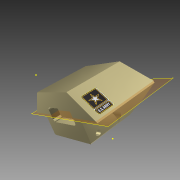
# Autodesk Inventor part: Correct BACK PIECE
Saved by Autodesk Inventor 2015 (Build 190159000, 159)
## iProperties
Created: 2015-04-17
Part Number: Correct BACK PIECE
Material: Generic
Document SubType Name: Modeling
Designer: Simrun
Density: 1 g/cm^3
Appearance: Gold - Metal
Mass: 1012.93 g
Surface Area: 682.37 cm^2
Volume: 1012.93 cm^3
Author: Simrun
Autodesk Inventor part; units mm, degrees
ref_plane "YZ Plane" through (0, 0, 0) normal (1, 0, 0) x (0, 1, 0)
ref_plane "XZ Plane" through (0, 0, 0) normal (0, 1, 0) x (-1, 0, 0)
sketch "Sketch1" plane through (0, 0, 0) normal (0, 0, 1) x (1, 0, 0)
  line L0 (0, 0) -> (0, 77.724)
  line L1 (0, 77.724) -> (101.6, 77.724)
  line L2 (101.6, 77.724) -> (114.3, 38.862)
  line L3 (114.3, 38.862) -> (101.6, 17.4625)
  line L4 (101.6, 17.4625) -> (92.075, 7.9375)
  line L5 (92.075, 7.9375) -> (79.375, 0)
  line L6 (79.375, 0) -> (0, 0)
  dimension "d0" = 77.724
  dimension "d1" = 101.6
  constraints: 14 end point, 1 horizontal, 1 perpendicular, 1 vertical
  measures "d0" distance of L0.start L0.end
  measures "d1" distance of L0.end L1.end
extrude "Extrusion1" add sketch "Sketch1" against normal blind 171.45
chamfer "Chamfer1" distance 41.275 angle 45 1 edges at (50.8, 77.724, 0)
chamfer "Chamfer2" distance 36.449 angle 45 1 edges at (39.6875, 0, 0)
chamfer "Chamfer3" distance 41.275 angle 45 1 edges at (50.8, 77.724, -171.45)
chamfer "Chamfer4" distance 36.449 angle 45 1 edges at (39.6875, 0, -171.45)
ref_plane "Work Plane1" through (0, 122.174, -85.725) normal (0, 0, 1) x (1, 0, 0)
ref_plane "Work Plane2" through (0, 0, -35.052) normal (0, 0, 1) x (1, 0, 0)
sketch "Sketch2" plane through (0, 0, -35.052) normal (0, 0, 1) x (1, 0, 0)
  line L0 (0, 36.449) -> (0, 0) projected
  line L1 (0, 1.5875) -> (0, 36.5125)
  line L2 (0, 36.5125) -> (19.2786, 36.5125)
  line L3 (0, 0) -> (79.375, 0) projected
  arc A0 (54.1154, 0) -> (19.2786, 36.5125) centre (19.2786, 1.6373) ccw
  line L4 (0, 1.5875) -> (54.1538, 1.5875)
  dimension "d17" = 34.925
  dimension "d18" = 19.2786
  constraints: 6 end point, 3 point on circle, 2 point on line, 1 centre point, 1 collinear, 1 parallel, 1 perpendicular, 1 tangent
  measures "d17" distance of L1.start L1.end
  measures "d18" distance of L1.end L2.end
extrude "Extrusion2" add sketch "Sketch2" along normal blind 35.052 contours L1 L2 A0 L4 L0
sketch "Sketch3" plane through (0, 0, 0) normal (0, 0, 1) x (1, 0, 0)
  line L0 (0, 1.5875) -> (0, 36.5125)
  line L1 (0, 77.724) -> (0, 36.5125) projected
  line L2 (0, 36.5125) -> (19.2786, 36.5125)
  line L3 (0, 36.5125) -> (19.2786, 36.5125) projected
  arc A0 (55.5625, 1.5875) -> (19.2786, 36.5125) centre (20.2634, 1.2253) ccw
  line L4 (55.5625, 1.5875) -> (0, 1.5875)
  line L5 (0, 0) -> (79.375, 0) projected
  constraints: 6 end point, 2 collinear, 2 point on circle, 1 centre point, 1 parallel
extrude "Extrusion3" cut sketch "Sketch3" against normal blind 35.052
mirror "Mirror1" about plane through (0, 122.174, -85.725) normal (0, 0, 1) of "Extrusion3"
ref_plane "Work Plane3" through (112.868, 36.449, 0) normal (-0.0005626, -0.9999998, 0) x (-0.9999997, 0.0005626, -0.0005626)
sketch "Sketch4" plane through (0, 0, -35.052) normal (0, 0, 1) x (1, 0, 0)
  line L0 (55.5625, 1.5875) -> (16.6624, 1.5875)
  line L1 (55.5625, 1.5875) -> (0, 1.5875) projected
  line L2 (16.6624, 1.5875) -> (16.6624, 7.9375)
  circle A0 centre (16.6624, 7.9375) radius 4.572
  point P0 (0, 0)
  dimension "d23" = 38.9001
  dimension "d24" = 6.35
  dimension "d25" = 9.144
  constraints: 4 end point, 1 centre point, 1 coincident, 1 point on line, 1 vertical
  measures "d23" distance of L0.start L0.end
  measures "d24" distance of L0.end L2.end
  measures "d25" diameter of A0
extrude "Extrusion4" cut sketch "Sketch4" against normal blind 10.16
mirror "Mirror2" about plane through (0, 122.174, -85.725) normal (0, 0, 1) of "Extrusion4"
sketch "Sketch5" plane through (0, 77.724, -41.275) normal (0, 0.7071068, 0.7071068) x (1, 0, 0)
  line L0 (10.4166, -16.3549) -> (37.5444, -16.3549) construction
  line L1 (37.5444, -16.3549) -> (37.5444, -50.6938) construction
  line L2 (37.5444, -50.6938) -> (10.4166, -50.6938) construction
  line L3 (10.4166, -50.6938) -> (10.4166, -16.3549) construction
  point P0 (0, -84.145)
  constraints: 2 other
sketch "Sketch6" plane through (0, 77.724, -130.175) normal (-1, 0, 0) x (0, 0, 1)
  line L0 (12.7, -26.162) -> (76.2, -26.162)
  line L1 (76.2, -26.162) -> (76.2, -51.562)
  line L2 (76.2, -51.562) -> (12.7, -51.562)
  line L3 (12.7, -51.562) -> (12.7, -26.162)
  line L4 (95.123, -76.1365) -> (95.123, -41.2115) projected
  line L5 (88.9, 0) -> (0, 0) projected
  point P0 (130.175, -77.724)
  dimension "d44" = 63.5
  dimension "d45" = 25.4
  dimension "d46" = 18.923
  dimension "d47" = 26.162
  constraints: 8 end point, 2 horizontal, 2 perpendicular
  measures "d44" distance of L0.start L0.end
  measures "d45" distance of L0.end L1.end
  measures "d46" distance between parallel lines of L4 L1
  measures "d47" distance between parallel lines of L5 L0
extrude "Extrusion5" cut sketch "Sketch6" against normal blind 14.478
fillet "Fillet1" radius 5.08 4 edges at (7.239, 51.562, -117.475) (7.239, 51.562, -53.975) (7.239, 26.162, -117.475) (7.239, 26.162, -53.975)
ref_plane "Work Plane4" through (0, 38.862, -41.275) normal (0, 1, 0) x (1, 0, 0)
sketch "Sketch7" plane through (114.3, 38.862, -2.413) normal (0.9505306, 0.3106309, 0) x (0, 0, -1)
  line L0 (68.5999, 25.7598) -> (96.6605, 25.7598) construction
  line L1 (96.6605, 25.7598) -> (96.6605, 14.7456) construction
  line L2 (96.6605, 14.7456) -> (68.5999, 14.7456) construction
  line L3 (68.5999, 14.7456) -> (68.5999, 25.7598) construction
  line L4 (71.7776, 31.7341) -> (71.0108, 31.7341)
  line L5 (71.0108, 31.7341) -> (69.7861, 33.9468)
  line L6 (69.7861, 33.9468) -> (69.7861, 31.7341)
  line L7 (69.7861, 31.7341) -> (69.058, 31.7341)
  line L8 (69.058, 31.7341) -> (69.058, 34.9091)
  line L9 (69.058, 34.9091) -> (70.0357, 34.9091)
  line L10 (70.0357, 34.9091) -> (71.0494, 33.0901)
  line L11 (71.0494, 33.0901) -> (71.0494, 34.9091)
  line L12 (71.0494, 34.9091) -> (71.7776, 34.9091)
  line L13 (71.7776, 34.9091) -> (71.7776, 31.7341)
  line L14 (72.4234, 31.7341) -> (72.4234, 34.9091)
  line L15 (72.4234, 34.9091) -> (74.5692, 34.9091)
  line L16 (74.5692, 34.9091) -> (74.5692, 34.3045)
  line L17 (74.5692, 34.3045) -> (73.2158, 34.3045)
  line L18 (73.2158, 34.3045) -> (73.2158, 33.7462)
  line L19 (73.2158, 33.7462) -> (74.4637, 33.7462)
  line L20 (74.4637, 33.7462) -> (74.4637, 33.1415)
  line L21 (74.4637, 33.1415) -> (73.2158, 33.1415)
  line L22 (73.2158, 33.1415) -> (73.2158, 32.3388)
  line L23 (73.2158, 32.3388) -> (74.5692, 32.3388)
  line L24 (74.5692, 32.3388) -> (74.5692, 31.7341)
  line L25 (74.5692, 31.7341) -> (72.4234, 31.7341)
  line L26 (77.7596, 34.9091) -> (76.6687, 31.7341)
  line L27 (76.6687, 31.7341) -> (75.8377, 31.7341)
  line L28 (75.8377, 31.7341) -> (74.7467, 34.9091)
  line L29 (74.7467, 34.9091) -> (75.5726, 34.9091)
  line L30 (75.5726, 34.9091) -> (76.2648, 32.7556)
  line L31 (76.2648, 32.7556) -> (76.9543, 34.9091)
  line L32 (76.9543, 34.9091) -> (77.7596, 34.9091)
  line L33 (78.0555, 31.7341) -> (78.0555, 34.9091)
  line L34 (78.0555, 34.9091) -> (80.2014, 34.9091)
  line L35 (80.2014, 34.9091) -> (80.2014, 34.3045)
  line L36 (80.2014, 34.3045) -> (78.848, 34.3045)
  line L37 (78.848, 34.3045) -> (78.848, 33.7462)
  line L38 (78.848, 33.7462) -> (80.0959, 33.7462)
  line L39 (80.0959, 33.7462) -> (80.0959, 33.1415)
  line L40 (80.0959, 33.1415) -> (78.848, 33.1415)
  line L41 (78.848, 33.1415) -> (78.848, 32.3388)
  line L42 (78.848, 32.3388) -> (80.2014, 32.3388)
  line L43 (80.2014, 32.3388) -> (80.2014, 31.7341)
  line L44 (80.2014, 31.7341) -> (78.0555, 31.7341)
  line L45 (83.6748, 31.7341) -> (82.7048, 31.7341)
  line L46 (82.7048, 31.7341) -> (81.8223, 32.8997)
  line L47 (81.8223, 32.8997) -> (81.5341, 32.8997)
  line L48 (81.5341, 32.8997) -> (81.5341, 31.7341)
  line L49 (81.5341, 31.7341) -> (80.7417, 31.7341)
  line L50 (80.7417, 31.7341) -> (80.7417, 34.9091)
  line L51 (80.7417, 34.9091) -> (82.0178, 34.9091)
  spline S0 degree 2 poles (82.0178, 34.9091) (82.2829, 34.9091) (82.6739, 34.8422) (82.8412, 34.7393) knots 0 0 0 1 2 2 2
  spline S1 degree 2 poles (82.8412, 34.7393) (83.011, 34.6312) (83.2117, 34.2942) (83.2117, 34.0369) knots 0 0 0 1 2 2 2
  spline S2 degree 2 poles (83.2117, 34.0369) (83.2117, 33.6741) (82.8823, 33.2187) (82.607, 33.0849) knots 0 0 0 1 2 2 2
  line L52 (82.607, 33.0849) -> (83.6748, 31.7341)
  spline S3 degree 2 poles (82.3935, 33.9366) (82.3935, 34.0575) (82.3009, 34.2299) (82.1954, 34.2762) knots 0 0 0 1 2 2 2
  spline S4 degree 2 poles (82.1954, 34.2762) (82.1208, 34.3071) (81.9381, 34.3251) (81.8017, 34.3251) knots 0 0 0 1 2 2 2
  line L53 (81.8017, 34.3251) -> (81.5341, 34.3251)
  line L54 (81.5341, 34.3251) -> (81.5341, 33.4709)
  line L55 (81.5341, 33.4709) -> (81.7631, 33.4709)
  spline S5 degree 2 poles (81.7631, 33.4709) (81.9278, 33.4709) (82.1619, 33.512) (82.2417, 33.5763) knots 0 0 0 1 2 2 2
  spline S6 degree 2 poles (82.2417, 33.5763) (82.3189, 33.6381) (82.3935, 33.8028) (82.3935, 33.9366) knots 0 0 0 1 2 2 2
  spline S7 degree 2 poles (86.1706, 31.6775) (85.8052, 31.6775) (85.2546, 31.819) (85.0179, 31.9219) knots 0 0 0 1 2 2 2
  line L56 (85.0179, 31.9219) -> (85.0179, 32.6784)
  line L57 (85.0179, 32.6784) -> (85.0899, 32.6784)
  spline S8 degree 2 poles (85.0899, 32.6784) (85.3292, 32.4751) (85.903, 32.2564) (86.1731, 32.2564) knots 0 0 0 1 2 2 2
  spline S9 degree 2 poles (86.1731, 32.2564) (86.2426, 32.2564) (86.4664, 32.2873) (86.5333, 32.3182) knots 0 0 0 1 2 2 2
  spline S10 degree 2 poles (86.5333, 32.3182) (86.6157, 32.3542) (86.7315, 32.4854) (86.7315, 32.5909) knots 0 0 0 1 2 2 2
  spline S11 degree 2 poles (86.7315, 32.5909) (86.7315, 32.7118) (86.5436, 32.8611) (86.415, 32.8945) knots 0 0 0 1 2 2 2
  spline S12 degree 2 poles (86.415, 32.8945) (86.2529, 32.9383) (85.885, 33.0129) (85.7229, 33.0695) knots 0 0 0 1 2 2 2
  spline S13 degree 2 poles (85.7229, 33.0695) (85.3549, 33.1981) (85.0359, 33.6381) (85.0359, 33.9674) knots 0 0 0 1 2 2 2
  spline S14 degree 2 poles (85.0359, 33.9674) (85.0359, 34.4125) (85.7898, 34.9657) (86.3558, 34.9657) knots 0 0 0 1 2 2 2
  spline S15 degree 2 poles (86.3558, 34.9657) (86.6388, 34.9657) (87.1997, 34.8499) (87.421, 34.7522) knots 0 0 0 1 2 2 2
  line L58 (87.421, 34.7522) -> (87.421, 34.0266)
  line L59 (87.421, 34.0266) -> (87.3515, 34.0266)
  spline S16 degree 2 poles (87.3515, 34.0266) (87.174, 34.1784) (86.6646, 34.3868) (86.397, 34.3868) knots 0 0 0 1 2 2 2
  spline S17 degree 2 poles (86.397, 34.3868) (86.2915, 34.3868) (86.1268, 34.3559) (86.0342, 34.3148) knots 0 0 0 1 2 2 2
  spline S18 degree 2 poles (86.0342, 34.3148) (85.9596, 34.2813) (85.8515, 34.1475) (85.8515, 34.0652) knots 0 0 0 1 2 2 2
  spline S19 degree 2 poles (85.8515, 34.0652) (85.8515, 33.9417) (86.0239, 33.8002) (86.2709, 33.7436) knots 0 0 0 1 2 2 2
  spline S20 degree 2 poles (86.2709, 33.7436) (86.4304, 33.7076) (86.7263, 33.6381) (86.8961, 33.5789) knots 0 0 0 1 2 2 2
  spline S21 degree 2 poles (86.8961, 33.5789) (87.2255, 33.458) (87.5471, 33.0566) (87.5471, 32.7273) knots 0 0 0 1 2 2 2
  spline S22 degree 2 poles (87.5471, 32.7273) (87.5471, 32.2539) (86.8035, 31.6775) (86.1706, 31.6775) knots 0 0 0 1 2 2 2
  line L60 (88.566, 31.7341) -> (88.566, 34.3045)
  line L61 (88.566, 34.3045) -> (87.6268, 34.3045)
  line L62 (87.6268, 34.3045) -> (87.6268, 34.9091)
  line L63 (87.6268, 34.9091) -> (90.3027, 34.9091)
  line L64 (90.3027, 34.9091) -> (90.3027, 34.3045)
  line L65 (90.3027, 34.3045) -> (89.3636, 34.3045)
  line L66 (89.3636, 34.3045) -> (89.3636, 31.7341)
  line L67 (89.3636, 31.7341) -> (88.566, 31.7341)
  spline S23 degree 2 poles (93.5189, 33.3216) (93.5189, 32.5497) (92.6955, 31.6672) (91.9802, 31.6672) knots 0 0 0 1 2 2 2
  spline S24 degree 2 poles (91.9802, 31.6672) (91.2624, 31.6672) (90.4442, 32.56) (90.4442, 33.3216) knots 0 0 0 1 2 2 2
  spline S25 degree 2 poles (90.4442, 33.3216) (90.4442, 34.0858) (91.2624, 34.976) (91.9802, 34.976) knots 0 0 0 1 2 2 2
  spline S26 degree 2 poles (91.9802, 34.976) (92.6955, 34.976) (93.5189, 34.0909) (93.5189, 33.3216) knots 0 0 0 1 2 2 2
  spline S27 degree 2 poles (92.6955, 33.3216) (92.6955, 33.6072) (92.5797, 34.006) (92.4794, 34.1321) knots 0 0 0 1 2 2 2
  spline S28 degree 2 poles (92.4794, 34.1321) (92.379, 34.2633) (92.1218, 34.3765) (91.9828, 34.3765) knots 0 0 0 1 2 2 2
  spline S29 degree 2 poles (91.9828, 34.3765) (91.8362, 34.3765) (91.5969, 34.271) (91.4862, 34.1372) knots 0 0 0 1 2 2 2
  spline S30 degree 2 poles (91.4862, 34.1372) (91.3885, 34.0137) (91.2675, 33.6046) (91.2675, 33.3216) knots 0 0 0 1 2 2 2
  spline S31 degree 2 poles (91.2675, 33.3216) (91.2675, 33.0283) (91.3833, 32.6424) (91.4837, 32.5111) knots 0 0 0 1 2 2 2
  spline S32 degree 2 poles (91.4837, 32.5111) (91.584, 32.3799) (91.8439, 32.2667) (91.9828, 32.2667) knots 0 0 0 1 2 2 2
  spline S33 degree 2 poles (91.9828, 32.2667) (92.1243, 32.2667) (92.3868, 32.3876) (92.482, 32.5163) knots 0 0 0 1 2 2 2
  spline S34 degree 2 poles (92.482, 32.5163) (92.5849, 32.6552) (92.6955, 33.0232) (92.6955, 33.3216) knots 0 0 0 1 2 2 2
  spline S35 degree 2 poles (96.434, 33.9082) (96.434, 33.687) (96.2925, 33.2856) (96.1613, 33.1518) knots 0 0 0 1 2 2 2
  spline S36 degree 2 poles (96.1613, 33.1518) (96.0815, 33.0669) (95.886, 32.928) (95.7702, 32.8791) knots 0 0 0 1 2 2 2
  spline S37 degree 2 poles (95.7702, 32.8791) (95.6518, 32.8302) (95.3765, 32.7736) (95.2067, 32.7736) knots 0 0 0 1 2 2 2
  line L68 (95.2067, 32.7736) -> (94.7899, 32.7736)
  line L69 (94.7899, 32.7736) -> (94.7899, 31.7341)
  line L70 (94.7899, 31.7341) -> (93.9923, 31.7341)
  line L71 (93.9923, 31.7341) -> (93.9923, 34.9091)
  line L72 (93.9923, 34.9091) -> (95.2247, 34.9091)
  spline S38 degree 2 poles (95.2247, 34.9091) (95.4974, 34.9091) (95.8962, 34.8088) (96.0583, 34.7007) knots 0 0 0 1 2 2 2
  spline S39 degree 2 poles (96.0583, 34.7007) (96.2384, 34.5798) (96.434, 34.1836) (96.434, 33.9082) knots 0 0 0 1 2 2 2
  spline S40 degree 2 poles (95.6158, 33.8877) (95.6158, 34.024) (95.4872, 34.217) (95.3997, 34.253) knots 0 0 0 1 2 2 2
  spline S41 degree 2 poles (95.3997, 34.253) (95.2865, 34.3019) (95.0806, 34.3173) (94.9031, 34.3173) knots 0 0 0 1 2 2 2
  line L73 (94.9031, 34.3173) -> (94.7899, 34.3173)
  line L74 (94.7899, 34.3173) -> (94.7899, 33.3654)
  line L75 (94.7899, 33.3654) -> (94.8465, 33.3654)
  spline S42 degree 2 poles (94.8465, 33.3654) (94.9571, 33.3654) (95.1578, 33.3705) (95.2324, 33.3834) knots 0 0 0 1 2 2 2
  spline S43 degree 2 poles (95.2324, 33.3834) (95.2968, 33.3937) (95.4383, 33.4554) (95.4769, 33.494) knots 0 0 0 1 2 2 2
  spline S44 degree 2 poles (95.4769, 33.494) (95.5592, 33.5712) (95.6158, 33.7436) (95.6158, 33.8877) knots 0 0 0 1 2 2 2
  line L76 (78.2524, 21.279) -> (77.4856, 21.279)
  line L77 (77.4856, 21.279) -> (76.2609, 23.4917)
  line L78 (76.2609, 23.4917) -> (76.2609, 21.279)
  line L79 (76.2609, 21.279) -> (75.5328, 21.279)
  line L80 (75.5328, 21.279) -> (75.5328, 24.454)
  line L81 (75.5328, 24.454) -> (76.5105, 24.454)
  line L82 (76.5105, 24.454) -> (77.5242, 22.6349)
  line L83 (77.5242, 22.6349) -> (77.5242, 24.454)
  line L84 (77.5242, 24.454) -> (78.2524, 24.454)
  line L85 (78.2524, 24.454) -> (78.2524, 21.279)
  line L86 (78.8982, 21.279) -> (78.8982, 24.454)
  line L87 (78.8982, 24.454) -> (81.044, 24.454)
  line L88 (81.044, 24.454) -> (81.044, 23.8494)
  line L89 (81.044, 23.8494) -> (79.6906, 23.8494)
  line L90 (79.6906, 23.8494) -> (79.6906, 23.291)
  line L91 (79.6906, 23.291) -> (80.9385, 23.291)
  line L92 (80.9385, 23.291) -> (80.9385, 22.6864)
  line L93 (80.9385, 22.6864) -> (79.6906, 22.6864)
  line L94 (79.6906, 22.6864) -> (79.6906, 21.8837)
  line L95 (79.6906, 21.8837) -> (81.044, 21.8837)
  line L96 (81.044, 21.8837) -> (81.044, 21.279)
  line L97 (81.044, 21.279) -> (78.8982, 21.279)
  line L98 (84.2344, 24.454) -> (83.1435, 21.279)
  line L99 (83.1435, 21.279) -> (82.3124, 21.279)
  line L100 (82.3124, 21.279) -> (81.2215, 24.454)
  line L101 (81.2215, 24.454) -> (82.0474, 24.454)
  line L102 (82.0474, 24.454) -> (82.7396, 22.3005)
  line L103 (82.7396, 22.3005) -> (83.4291, 24.454)
  line L104 (83.4291, 24.454) -> (84.2344, 24.454)
  line L105 (84.5303, 21.279) -> (84.5303, 24.454)
  line L106 (84.5303, 24.454) -> (86.6761, 24.454)
  line L107 (86.6761, 24.454) -> (86.6761, 23.8494)
  line L108 (86.6761, 23.8494) -> (85.3228, 23.8494)
  line L109 (85.3228, 23.8494) -> (85.3228, 23.291)
  line L110 (85.3228, 23.291) -> (86.5706, 23.291)
  line L111 (86.5706, 23.291) -> (86.5706, 22.6864)
  line L112 (86.5706, 22.6864) -> (85.3228, 22.6864)
  line L113 (85.3228, 22.6864) -> (85.3228, 21.8837)
  line L114 (85.3228, 21.8837) -> (86.6761, 21.8837)
  line L115 (86.6761, 21.8837) -> (86.6761, 21.279)
  line L116 (86.6761, 21.279) -> (84.5303, 21.279)
  line L117 (90.1496, 21.279) -> (89.1796, 21.279)
  line L118 (89.1796, 21.279) -> (88.2971, 22.4446)
  line L119 (88.2971, 22.4446) -> (88.0089, 22.4446)
  line L120 (88.0089, 22.4446) -> (88.0089, 21.279)
  line L121 (88.0089, 21.279) -> (87.2165, 21.279)
  line L122 (87.2165, 21.279) -> (87.2165, 24.454)
  line L123 (87.2165, 24.454) -> (88.4926, 24.454)
  spline S45 degree 2 poles (88.4926, 24.454) (88.7576, 24.454) (89.1487, 24.3871) (89.316, 24.2842) knots 0 0 0 1 2 2 2
  spline S46 degree 2 poles (89.316, 24.2842) (89.4858, 24.1761) (89.6865, 23.8391) (89.6865, 23.5818) knots 0 0 0 1 2 2 2
  spline S47 degree 2 poles (89.6865, 23.5818) (89.6865, 23.219) (89.3571, 22.7636) (89.0818, 22.6298) knots 0 0 0 1 2 2 2
  line L124 (89.0818, 22.6298) -> (90.1496, 21.279)
  spline S48 degree 2 poles (88.8683, 23.4814) (88.8683, 23.6024) (88.7757, 23.7748) (88.6702, 23.8211) knots 0 0 0 1 2 2 2
  spline S49 degree 2 poles (88.6702, 23.8211) (88.5955, 23.8519) (88.4129, 23.87) (88.2765, 23.87) knots 0 0 0 1 2 2 2
  line L125 (88.2765, 23.87) -> (88.0089, 23.87)
  line L126 (88.0089, 23.87) -> (88.0089, 23.0157)
  line L127 (88.0089, 23.0157) -> (88.2379, 23.0157)
  spline S50 degree 2 poles (88.2379, 23.0157) (88.4026, 23.0157) (88.6367, 23.0569) (88.7165, 23.1212) knots 0 0 0 1 2 2 2
  spline S51 degree 2 poles (88.7165, 23.1212) (88.7937, 23.183) (88.8683, 23.3477) (88.8683, 23.4814) knots 0 0 0 1 2 2 2
  spline S52 degree 2 poles (75.3089, 15.9949) (74.9436, 15.9949) (74.393, 16.1364) (74.1562, 16.2393) knots 0 0 0 1 2 2 2
  line L128 (74.1562, 16.2393) -> (74.1562, 16.9957)
  line L129 (74.1562, 16.9957) -> (74.2283, 16.9957)
  spline S53 degree 2 poles (74.2283, 16.9957) (74.4676, 16.7925) (75.0413, 16.5738) (75.3115, 16.5738) knots 0 0 0 1 2 2 2
  spline S54 degree 2 poles (75.3115, 16.5738) (75.381, 16.5738) (75.6048, 16.6046) (75.6717, 16.6355) knots 0 0 0 1 2 2 2
  spline S55 degree 2 poles (75.6717, 16.6355) (75.754, 16.6715) (75.8698, 16.8028) (75.8698, 16.9082) knots 0 0 0 1 2 2 2
  spline S56 degree 2 poles (75.8698, 16.9082) (75.8698, 17.0292) (75.682, 17.1784) (75.5533, 17.2119) knots 0 0 0 1 2 2 2
  spline S57 degree 2 poles (75.5533, 17.2119) (75.3913, 17.2556) (75.0233, 17.3302) (74.8612, 17.3868) knots 0 0 0 1 2 2 2
  spline S58 degree 2 poles (74.8612, 17.3868) (74.4933, 17.5155) (74.1743, 17.9554) (74.1743, 18.2848) knots 0 0 0 1 2 2 2
  spline S59 degree 2 poles (74.1743, 18.2848) (74.1743, 18.7299) (74.9281, 19.2831) (75.4942, 19.2831) knots 0 0 0 1 2 2 2
  spline S60 degree 2 poles (75.4942, 19.2831) (75.7772, 19.2831) (76.3381, 19.1673) (76.5594, 19.0695) knots 0 0 0 1 2 2 2
  line L130 (76.5594, 19.0695) -> (76.5594, 18.3439)
  line L131 (76.5594, 18.3439) -> (76.4899, 18.3439)
  spline S61 degree 2 poles (76.4899, 18.3439) (76.3124, 18.4957) (75.8029, 18.7042) (75.5353, 18.7042) knots 0 0 0 1 2 2 2
  spline S62 degree 2 poles (75.5353, 18.7042) (75.4298, 18.7042) (75.2652, 18.6733) (75.1726, 18.6321) knots 0 0 0 1 2 2 2
  spline S63 degree 2 poles (75.1726, 18.6321) (75.0979, 18.5987) (74.9899, 18.4649) (74.9899, 18.3825) knots 0 0 0 1 2 2 2
  spline S64 degree 2 poles (74.9899, 18.3825) (74.9899, 18.259) (75.1623, 18.1175) (75.4093, 18.0609) knots 0 0 0 1 2 2 2
  spline S65 degree 2 poles (75.4093, 18.0609) (75.5688, 18.0249) (75.8647, 17.9554) (76.0345, 17.8963) knots 0 0 0 1 2 2 2
  spline S66 degree 2 poles (76.0345, 17.8963) (76.3638, 17.7753) (76.6854, 17.3739) (76.6854, 17.0446) knots 0 0 0 1 2 2 2
  spline S67 degree 2 poles (76.6854, 17.0446) (76.6854, 16.5712) (75.9419, 15.9949) (75.3089, 15.9949) knots 0 0 0 1 2 2 2
  line L132 (77.0945, 16.0515) -> (77.0945, 19.2265)
  line L133 (77.0945, 19.2265) -> (79.2404, 19.2265)
  line L134 (79.2404, 19.2265) -> (79.2404, 18.6218)
  line L135 (79.2404, 18.6218) -> (77.887, 18.6218)
  line L136 (77.887, 18.6218) -> (77.887, 18.0635)
  line L137 (77.887, 18.0635) -> (79.1349, 18.0635)
  line L138 (79.1349, 18.0635) -> (79.1349, 17.4589)
  line L139 (79.1349, 17.4589) -> (77.887, 17.4589)
  line L140 (77.887, 17.4589) -> (77.887, 16.6561)
  line L141 (77.887, 16.6561) -> (79.2404, 16.6561)
  line L142 (79.2404, 16.6561) -> (79.2404, 16.0515)
  line L143 (79.2404, 16.0515) -> (77.0945, 16.0515)
  line L144 (80.3905, 16.0515) -> (80.3905, 18.6218)
  line L145 (80.3905, 18.6218) -> (79.4513, 18.6218)
  line L146 (79.4513, 18.6218) -> (79.4513, 19.2265)
  line L147 (79.4513, 19.2265) -> (82.1272, 19.2265)
  line L148 (82.1272, 19.2265) -> (82.1272, 18.6218)
  line L149 (82.1272, 18.6218) -> (81.1881, 18.6218)
  line L150 (81.1881, 18.6218) -> (81.1881, 16.0515)
  line L151 (81.1881, 16.0515) -> (80.3905, 16.0515)
  line L152 (83.0637, 16.0515) -> (83.0637, 18.6218)
  line L153 (83.0637, 18.6218) -> (82.1246, 18.6218)
  line L154 (82.1246, 18.6218) -> (82.1246, 19.2265)
  line L155 (82.1246, 19.2265) -> (84.8005, 19.2265)
  line L156 (84.8005, 19.2265) -> (84.8005, 18.6218)
  line L157 (84.8005, 18.6218) -> (83.8614, 18.6218)
  line L158 (83.8614, 18.6218) -> (83.8614, 16.0515)
  line L159 (83.8614, 16.0515) -> (83.0637, 16.0515)
  line L160 (87.2448, 16.0515) -> (85.1272, 16.0515)
  line L161 (85.1272, 16.0515) -> (85.1272, 19.2265)
  line L162 (85.1272, 19.2265) -> (85.9248, 19.2265)
  line L163 (85.9248, 19.2265) -> (85.9248, 16.6561)
  line L164 (85.9248, 16.6561) -> (87.2448, 16.6561)
  line L165 (87.2448, 16.6561) -> (87.2448, 16.0515)
  line L166 (87.6256, 16.0515) -> (87.6256, 19.2265)
  line L167 (87.6256, 19.2265) -> (89.7714, 19.2265)
  line L168 (89.7714, 19.2265) -> (89.7714, 18.6218)
  line L169 (89.7714, 18.6218) -> (88.418, 18.6218)
  line L170 (88.418, 18.6218) -> (88.418, 18.0635)
  line L171 (88.418, 18.0635) -> (89.6659, 18.0635)
  line L172 (89.6659, 18.0635) -> (89.6659, 17.4589)
  line L173 (89.6659, 17.4589) -> (88.418, 17.4589)
  line L174 (88.418, 17.4589) -> (88.418, 16.6561)
  line L175 (88.418, 16.6561) -> (89.7714, 16.6561)
  line L176 (89.7714, 16.6561) -> (89.7714, 16.0515)
  line L177 (89.7714, 16.0515) -> (87.6256, 16.0515)
  spline S68 degree 2 poles (72.579, 5.5295) (71.9384, 5.5295) (71.2488, 6.147) (71.2488, 6.7439) knots 0 0 0 1 2 2 2
  line L178 (71.2488, 6.7439) -> (71.2488, 8.7714)
  line L179 (71.2488, 8.7714) -> (72.0464, 8.7714)
  line L180 (72.0464, 8.7714) -> (72.0464, 6.7902)
  spline S69 degree 2 poles (72.0464, 6.7902) (72.0464, 6.4583) (72.296, 6.1341) (72.579, 6.1341) knots 0 0 0 1 2 2 2
  spline S70 degree 2 poles (72.579, 6.1341) (72.8543, 6.1341) (73.1116, 6.4454) (73.1116, 6.7902) knots 0 0 0 1 2 2 2
  line L181 (73.1116, 6.7902) -> (73.1116, 8.7714)
  line L182 (73.1116, 8.7714) -> (73.9092, 8.7714)
  line L183 (73.9092, 8.7714) -> (73.9092, 6.7465)
  spline S71 degree 2 poles (73.9092, 6.7465) (73.9092, 6.1598) (73.2377, 5.5295) (72.579, 5.5295) knots 0 0 0 1 2 2 2
  spline S72 degree 2 poles (75.5019, 5.5397) (75.1365, 5.5397) (74.5859, 5.6813) (74.3492, 5.7842) knots 0 0 0 1 2 2 2
  line L184 (74.3492, 5.7842) -> (74.3492, 6.5406)
  line L185 (74.3492, 6.5406) -> (74.4213, 6.5406)
  spline S73 degree 2 poles (74.4213, 6.5406) (74.6605, 6.3374) (75.2343, 6.1187) (75.5045, 6.1187) knots 0 0 0 1 2 2 2
  spline S74 degree 2 poles (75.5045, 6.1187) (75.5739, 6.1187) (75.7978, 6.1495) (75.8647, 6.1804) knots 0 0 0 1 2 2 2
  spline S75 degree 2 poles (75.8647, 6.1804) (75.947, 6.2164) (76.0628, 6.3476) (76.0628, 6.4531) knots 0 0 0 1 2 2 2
  spline S76 degree 2 poles (76.0628, 6.4531) (76.0628, 6.5741) (75.875, 6.7233) (75.7463, 6.7567) knots 0 0 0 1 2 2 2
  spline S77 degree 2 poles (75.7463, 6.7567) (75.5842, 6.8005) (75.2163, 6.8751) (75.0542, 6.9317) knots 0 0 0 1 2 2 2
  spline S78 degree 2 poles (75.0542, 6.9317) (74.6863, 7.0604) (74.3672, 7.5003) (74.3672, 7.8297) knots 0 0 0 1 2 2 2
  spline S79 degree 2 poles (74.3672, 7.8297) (74.3672, 8.2748) (75.1211, 8.828) (75.6871, 8.828) knots 0 0 0 1 2 2 2
  spline S80 degree 2 poles (75.6871, 8.828) (75.9702, 8.828) (76.5311, 8.7122) (76.7523, 8.6144) knots 0 0 0 1 2 2 2
  line L186 (76.7523, 8.6144) -> (76.7523, 7.8888)
  line L187 (76.7523, 7.8888) -> (76.6829, 7.8888)
  spline S81 degree 2 poles (76.6829, 7.8888) (76.5053, 8.0406) (75.9959, 8.249) (75.7283, 8.249) knots 0 0 0 1 2 2 2
  spline S82 degree 2 poles (75.7283, 8.249) (75.6228, 8.249) (75.4581, 8.2182) (75.3655, 8.177) knots 0 0 0 1 2 2 2
  spline S83 degree 2 poles (75.3655, 8.177) (75.2909, 8.1436) (75.1828, 8.0098) (75.1828, 7.9274) knots 0 0 0 1 2 2 2
  spline S84 degree 2 poles (75.1828, 7.9274) (75.1828, 7.8039) (75.3552, 7.6624) (75.6022, 7.6058) knots 0 0 0 1 2 2 2
  spline S85 degree 2 poles (75.6022, 7.6058) (75.7618, 7.5698) (76.0576, 7.5003) (76.2275, 7.4411) knots 0 0 0 1 2 2 2
  spline S86 degree 2 poles (76.2275, 7.4411) (76.5568, 7.3202) (76.8784, 6.9188) (76.8784, 6.5895) knots 0 0 0 1 2 2 2
  spline S87 degree 2 poles (76.8784, 6.5895) (76.8784, 6.1161) (76.1348, 5.5397) (75.5019, 5.5397) knots 0 0 0 1 2 2 2
  line L188 (76.9453, 5.5964) -> (78.0182, 8.7714)
  line L189 (78.0182, 8.7714) -> (78.8879, 8.7714)
  line L190 (78.8879, 8.7714) -> (79.9608, 5.5964)
  line L191 (79.9608, 5.5964) -> (79.14, 5.5964)
  line L192 (79.14, 5.5964) -> (78.9419, 6.2447)
  line L193 (78.9419, 6.2447) -> (77.9436, 6.2447)
  line L194 (77.9436, 6.2447) -> (77.7429, 5.5964)
  line L195 (77.7429, 5.5964) -> (76.9453, 5.5964)
  line L196 (78.7669, 6.8211) -> (78.4428, 7.8708)
  line L197 (78.4428, 7.8708) -> (78.116, 6.8211)
  line L198 (78.116, 6.8211) -> (78.7669, 6.8211)
  line L199 (81.2138, 5.5964) -> (82.2867, 8.7714)
  line L200 (82.2867, 8.7714) -> (83.1564, 8.7714)
  line L201 (83.1564, 8.7714) -> (84.2293, 5.5964)
  line L202 (84.2293, 5.5964) -> (83.4085, 5.5964)
  line L203 (83.4085, 5.5964) -> (83.2104, 6.2447)
  line L204 (83.2104, 6.2447) -> (82.2121, 6.2447)
  line L205 (82.2121, 6.2447) -> (82.0114, 5.5964)
  line L206 (82.0114, 5.5964) -> (81.2138, 5.5964)
  line L207 (83.0354, 6.8211) -> (82.7112, 7.8708)
  line L208 (82.7112, 7.8708) -> (82.3845, 6.8211)
  line L209 (82.3845, 6.8211) -> (83.0354, 6.8211)
  line L210 (87.4789, 5.5964) -> (86.5089, 5.5964)
  line L211 (86.5089, 5.5964) -> (85.6264, 6.7619)
  line L212 (85.6264, 6.7619) -> (85.3382, 6.7619)
  line L213 (85.3382, 6.7619) -> (85.3382, 5.5964)
  line L214 (85.3382, 5.5964) -> (84.5458, 5.5964)
  line L215 (84.5458, 5.5964) -> (84.5458, 8.7714)
  line L216 (84.5458, 8.7714) -> (85.8219, 8.7714)
  spline S88 degree 2 poles (85.8219, 8.7714) (86.0869, 8.7714) (86.478, 8.7045) (86.6453, 8.6015) knots 0 0 0 1 2 2 2
  spline S89 degree 2 poles (86.6453, 8.6015) (86.8151, 8.4935) (87.0158, 8.1564) (87.0158, 7.8991) knots 0 0 0 1 2 2 2
  spline S90 degree 2 poles (87.0158, 7.8991) (87.0158, 7.5363) (86.6864, 7.0809) (86.4111, 6.9471) knots 0 0 0 1 2 2 2
  line L217 (86.4111, 6.9471) -> (87.4789, 5.5964)
  spline S91 degree 2 poles (86.1976, 7.7988) (86.1976, 7.9197) (86.1049, 8.0921) (85.9995, 8.1384) knots 0 0 0 1 2 2 2
  spline S92 degree 2 poles (85.9995, 8.1384) (85.9248, 8.1693) (85.7422, 8.1873) (85.6058, 8.1873) knots 0 0 0 1 2 2 2
  line L218 (85.6058, 8.1873) -> (85.3382, 8.1873)
  line L219 (85.3382, 8.1873) -> (85.3382, 7.3331)
  line L220 (85.3382, 7.3331) -> (85.5672, 7.3331)
  spline S93 degree 2 poles (85.5672, 7.3331) (85.7319, 7.3331) (85.966, 7.3742) (86.0458, 7.4386) knots 0 0 0 1 2 2 2
  spline S94 degree 2 poles (86.0458, 7.4386) (86.123, 7.5003) (86.1976, 7.665) (86.1976, 7.7988) knots 0 0 0 1 2 2 2
  line L221 (90.9575, 5.5964) -> (90.165, 5.5964)
  line L222 (90.165, 5.5964) -> (90.165, 7.701)
  line L223 (90.165, 7.701) -> (89.5887, 6.3425)
  line L224 (89.5887, 6.3425) -> (89.0432, 6.3425)
  line L225 (89.0432, 6.3425) -> (88.4669, 7.701)
  line L226 (88.4669, 7.701) -> (88.4669, 5.5964)
  line L227 (88.4669, 5.5964) -> (87.7156, 5.5964)
  line L228 (87.7156, 5.5964) -> (87.7156, 8.7714)
  line L229 (87.7156, 8.7714) -> (88.6341, 8.7714)
  line L230 (88.6341, 8.7714) -> (89.3391, 7.2044)
  line L231 (89.3391, 7.2044) -> (90.039, 8.7714)
  line L232 (90.039, 8.7714) -> (90.9575, 8.7714)
  line L233 (90.9575, 8.7714) -> (90.9575, 5.5964)
  line L234 (94.256, 8.7714) -> (93.1599, 6.9214)
  line L235 (93.1599, 6.9214) -> (93.1599, 5.5964)
  line L236 (93.1599, 5.5964) -> (92.3623, 5.5964)
  line L237 (92.3623, 5.5964) -> (92.3623, 6.8828)
  line L238 (92.3623, 6.8828) -> (91.2482, 8.7714)
  line L239 (91.2482, 8.7714) -> (92.1565, 8.7714)
  line L240 (92.1565, 8.7714) -> (92.7766, 7.6393)
  line L241 (92.7766, 7.6393) -> (93.3761, 8.7714)
  line L242 (93.3761, 8.7714) -> (94.256, 8.7714)
  point P0 (-2.413, -1.4344)
  constraints: 2 other
extrude "Extrusion6" add sketch "Sketch7" along normal blind 1.27
sketch "Sketch8" plane through (101.6, 77.724, -130.175) normal (0, 0.7071068, -0.7071068) x (-1, 0, 0)
  line L0 (6.35, -55.5625) -> (69.85, -55.5625)
  line L1 (69.85, -55.5625) -> (69.85, -11.1125)
  line L2 (69.85, -11.1125) -> (6.35, -11.1125)
  line L3 (6.35, -11.1125) -> (6.35, -55.5625)
  line L4 (38.1, -11.1125) -> (38.1, -55.5625)
  line L5 (6.35, -33.3375) -> (69.85, -33.3375)
  line L6 (6.35, -22.225) -> (69.85, -22.225)
  line L7 (6.35, -44.45) -> (69.85, -44.45)
  point P0 (101.6, 37.0885)
  constraints: 16 end point, 4 midpoint, 4 point on line, 3 perpendicular, 2 parallel, 1 horizontal
extrude "Extrusion7" add sketch "Sketch8" along normal blind 2.54
sketch "Sketch9" plane through (101.6, 79.5201, -131.9711) normal (0, 0.7071068, -0.7071068) x (-1, 0, 0)
  point P0 (101.6, 37.0885)
sketch "Sketch10" plane through (101.6, 79.5201, -131.9711) normal (0, 0.7071068, -0.7071068) x (-1, 0, 0)
  point P0 (101.6, 37.0885)
sketch "Sketch11" plane through (101.6, 79.5201, -131.9711) normal (0, 0.7071068, -0.7071068) x (-1, 0, 0)
  point P0 (101.6, 37.0885)
sketch "Sketch12" plane through (101.6, 79.5201, -131.9711) normal (0, 0.7071068, -0.7071068) x (-1, 0, 0)
  line L0 (6.35, -55.5625) -> (69.85, -55.5625) projected
  line L1 (69.85, -55.5625) -> (69.85, -11.1125) projected
  line L2 (69.85, -11.1125) -> (6.35, -11.1125) projected
  line L3 (6.35, -11.1125) -> (6.35, -55.5625) projected
  line L4 (65.0875, -26.9875) -> (61.9125, -26.9875)
  line L5 (61.9125, -26.9875) -> (61.9125, -44.45)
  line L6 (61.9125, -44.45) -> (65.0875, -44.45)
  line L7 (65.0875, -44.45) -> (65.0875, -26.9875)
  point P0 (101.6, 37.0885)
  constraints: 8 end point, 2 parallel, 1 horizontal, 1 perpendicular
extrude "Extrusion8" add sketch "Sketch12" along normal blind 2.54 contours L7 L6 L5 L4
sketch "Sketch13" plane through (79.375, 0, -135.001) normal (0, -0.7071068, -0.7071068) x (-1, 0, 0)
  line L0 (-12.8127, 50.591) -> (0.1104, 50.591) construction
  line L1 (0.1104, 50.591) -> (0.1104, 14.3843) construction
  line L2 (0.1104, 14.3843) -> (-12.8127, 14.3843) construction
  line L3 (-12.8127, 14.3843) -> (-12.8127, 50.591) construction
  line L4 (-10.071, 44.495) -> (-12.4323, 44.495)
  line L5 (-12.4323, 44.495) -> (-12.4323, 45.1175)
  line L6 (-12.4323, 45.1175) -> (-11.6567, 45.1175)
  line L7 (-11.6567, 45.1175) -> (-11.6567, 49.9686)
  line L8 (-11.6567, 49.9686) -> (-12.4323, 49.9686)
  line L9 (-12.4323, 49.9686) -> (-12.4323, 50.591)
  line L10 (-12.4323, 50.591) -> (-10.071, 50.591)
  line L11 (-10.071, 50.591) -> (-10.071, 49.9686)
  line L12 (-10.071, 49.9686) -> (-10.8466, 49.9686)
  line L13 (-10.8466, 49.9686) -> (-10.8466, 45.1175)
  line L14 (-10.8466, 45.1175) -> (-10.071, 45.1175)
  line L15 (-10.071, 45.1175) -> (-10.071, 44.495)
  line L16 (-2.2361, 50.591) -> (-3.7675, 44.495)
  line L17 (-3.7675, 44.495) -> (-4.6765, 44.495)
  line L18 (-4.6765, 44.495) -> (-5.9164, 49.5536)
  line L19 (-5.9164, 49.5536) -> (-7.1218, 44.495)
  line L20 (-7.1218, 44.495) -> (-8.0209, 44.495)
  line L21 (-8.0209, 44.495) -> (-9.577, 50.591)
  line L22 (-9.577, 50.591) -> (-8.7421, 50.591)
  line L23 (-8.7421, 50.591) -> (-7.517, 45.5374)
  line L24 (-7.517, 45.5374) -> (-6.3017, 50.591)
  line L25 (-6.3017, 50.591) -> (-5.4768, 50.591)
  line L26 (-5.4768, 50.591) -> (-4.2516, 45.4781)
  line L27 (-4.2516, 45.4781) -> (-3.0314, 50.591)
  line L28 (-3.0314, 50.591) -> (-2.2361, 50.591)
  line L29 (-6.9687, 34.4581) -> (-7.7788, 34.4581)
  line L30 (-7.7788, 34.4581) -> (-7.7788, 39.7094)
  line L31 (-7.7788, 39.7094) -> (-9.3695, 36.1378)
  line L32 (-9.3695, 36.1378) -> (-9.8635, 36.1378)
  line L33 (-9.8635, 36.1378) -> (-11.4394, 39.7094)
  line L34 (-11.4394, 39.7094) -> (-11.4394, 34.4581)
  line L35 (-11.4394, 34.4581) -> (-12.1952, 34.4581)
  line L36 (-12.1952, 34.4581) -> (-12.1952, 40.5541)
  line L37 (-12.1952, 40.5541) -> (-11.0886, 40.5541)
  line L38 (-11.0886, 40.5541) -> (-9.5671, 37.1603)
  line L39 (-9.5671, 37.1603) -> (-8.095, 40.5541)
  line L40 (-8.095, 40.5541) -> (-6.9687, 40.5541)
  line L41 (-6.9687, 40.5541) -> (-6.9687, 34.4581)
  line L42 (-0.5071, 34.4581) -> (-1.3173, 34.4581)
  line L43 (-1.3173, 34.4581) -> (-1.3173, 39.7094)
  line L44 (-1.3173, 39.7094) -> (-2.9079, 36.1378)
  line L45 (-2.9079, 36.1378) -> (-3.4019, 36.1378)
  line L46 (-3.4019, 36.1378) -> (-4.9778, 39.7094)
  line L47 (-4.9778, 39.7094) -> (-4.9778, 34.4581)
  line L48 (-4.9778, 34.4581) -> (-5.7336, 34.4581)
  line L49 (-5.7336, 34.4581) -> (-5.7336, 40.5541)
  line L50 (-5.7336, 40.5541) -> (-4.6271, 40.5541)
  line L51 (-4.6271, 40.5541) -> (-3.1055, 37.1603)
  line L52 (-3.1055, 37.1603) -> (-1.6334, 40.5541)
  line L53 (-1.6334, 40.5541) -> (-0.5071, 40.5541)
  line L54 (-0.5071, 40.5541) -> (-0.5071, 34.4581)
  line L55 (-12.8522, 24.4212) -> (-10.7972, 30.5172)
  line L56 (-10.7972, 30.5172) -> (-9.7993, 30.5172)
  line L57 (-9.7993, 30.5172) -> (-7.7442, 24.4212)
  line L58 (-7.7442, 24.4212) -> (-8.5989, 24.4212)
  line L59 (-8.5989, 24.4212) -> (-9.1521, 26.1256)
  line L60 (-9.1521, 26.1256) -> (-11.4789, 26.1256)
  line L61 (-11.4789, 26.1256) -> (-12.0322, 24.4212)
  line L62 (-12.0322, 24.4212) -> (-12.8522, 24.4212)
  line L63 (-9.3744, 26.8172) -> (-10.318, 29.6873)
  line L64 (-10.318, 29.6873) -> (-11.2566, 26.8172)
  line L65 (-11.2566, 26.8172) -> (-9.3744, 26.8172)
  spline S0 degree 2 poles (-5.4669, 24.3126) (-6.1288, 24.3126) (-7.0576, 24.5892) (-7.4676, 24.7868) knots 0 0 0 1 2 2 2
  line L66 (-7.4676, 24.7868) -> (-7.4676, 25.8044)
  line L67 (-7.4676, 25.8044) -> (-7.4083, 25.8044)
  spline S1 degree 2 poles (-7.4083, 25.8044) (-7.0082, 25.429) (-5.9955, 25.014) (-5.5262, 25.014) knots 0 0 0 1 2 2 2
  spline S2 degree 2 poles (-5.5262, 25.014) (-4.8543, 25.014) (-4.1677, 25.5723) (-4.1677, 26.0317) knots 0 0 0 1 2 2 2
  spline S3 degree 2 poles (-4.1677, 26.0317) (-4.1677, 26.3973) (-4.5283, 26.8517) (-4.9185, 26.9654) knots 0 0 0 1 2 2 2
  spline S4 degree 2 poles (-4.9185, 26.9654) (-5.2001, 27.0444) (-5.6694, 27.1531) (-6.0202, 27.242) knots 0 0 0 1 2 2 2
  spline S5 degree 2 poles (-6.0202, 27.242) (-6.3363, 27.326) (-6.8353, 27.5779) (-7.0279, 27.7805) knots 0 0 0 1 2 2 2
  spline S6 degree 2 poles (-7.0279, 27.7805) (-7.2157, 27.983) (-7.4231, 28.5264) (-7.4231, 28.8821) knots 0 0 0 1 2 2 2
  spline S7 degree 2 poles (-7.4231, 28.8821) (-7.4231, 29.6231) (-6.2672, 30.6259) (-5.373, 30.6259) knots 0 0 0 1 2 2 2
  spline S8 degree 2 poles (-5.373, 30.6259) (-4.8593, 30.6259) (-3.9503, 30.4234) (-3.56, 30.2307) knots 0 0 0 1 2 2 2
  line L68 (-3.56, 30.2307) -> (-3.56, 29.2625)
  line L69 (-3.56, 29.2625) -> (-3.6193, 29.2625)
  spline S9 degree 2 poles (-3.6193, 29.2625) (-3.9108, 29.5292) (-4.8197, 29.9244) (-5.3187, 29.9244) knots 0 0 0 1 2 2 2
  spline S10 degree 2 poles (-5.3187, 29.9244) (-5.8818, 29.9244) (-6.5784, 29.3959) (-6.5784, 28.9661) knots 0 0 0 1 2 2 2
  spline S11 degree 2 poles (-6.5784, 28.9661) (-6.5784, 28.5807) (-6.1684, 28.1213) (-5.783, 28.0176) knots 0 0 0 1 2 2 2
  spline S12 degree 2 poles (-5.783, 28.0176) (-5.5262, 27.9484) (-4.7802, 27.7706) (-4.5332, 27.6965) knots 0 0 0 1 2 2 2
  spline S13 degree 2 poles (-4.5332, 27.6965) (-3.9058, 27.5038) (-3.3229, 26.7282) (-3.3229, 26.1601) knots 0 0 0 1 2 2 2
  spline S14 degree 2 poles (-3.3229, 26.1601) (-3.3229, 25.7995) (-3.6144, 25.1079) (-3.8762, 24.8658) knots 0 0 0 1 2 2 2
  spline S15 degree 2 poles (-3.8762, 24.8658) (-4.1677, 24.5991) (-4.9087, 24.3126) (-5.4669, 24.3126) knots 0 0 0 1 2 2 2
  line L70 (-12.8522, 14.3843) -> (-10.7972, 20.4803)
  line L71 (-10.7972, 20.4803) -> (-9.7993, 20.4803)
  line L72 (-9.7993, 20.4803) -> (-7.7442, 14.3843)
  line L73 (-7.7442, 14.3843) -> (-8.5989, 14.3843)
  line L74 (-8.5989, 14.3843) -> (-9.1521, 16.0886)
  line L75 (-9.1521, 16.0886) -> (-11.4789, 16.0886)
  line L76 (-11.4789, 16.0886) -> (-12.0322, 14.3843)
  line L77 (-12.0322, 14.3843) -> (-12.8522, 14.3843)
  line L78 (-9.3744, 16.7803) -> (-10.318, 19.6504)
  line L79 (-10.318, 19.6504) -> (-11.2566, 16.7803)
  line L80 (-11.2566, 16.7803) -> (-9.3744, 16.7803)
  line L81 (-3.6341, 14.3843) -> (-7.1663, 14.3843)
  line L82 (-7.1663, 14.3843) -> (-7.1663, 20.4803)
  line L83 (-7.1663, 20.4803) -> (-6.3561, 20.4803)
  line L84 (-6.3561, 20.4803) -> (-6.3561, 15.1056)
  line L85 (-6.3561, 15.1056) -> (-3.6341, 15.1056)
  line L86 (-3.6341, 15.1056) -> (-3.6341, 14.3843)
  point P0 (79.375, -95.4601)
  constraints: 2 other
extrude "Extrusion9" add sketch "Sketch13" along normal blind 1.27
body "Solid1"
